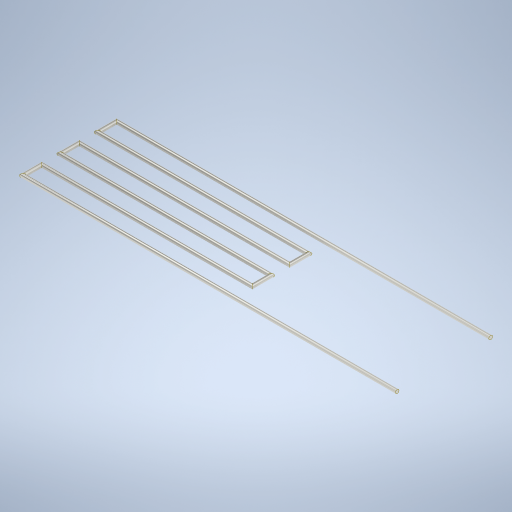
# Autodesk Inventor part: strain guage abs
Saved by Autodesk Inventor 2024.2 (Build 282272000, 272)
## iProperties
Created: 2024-07-17
Part Number: strain guage abs
Material: Silver
Document SubType Name: Modeling
Designer: Makerspace
Density: 10.49 g/cm^3
Appearance: Silver
Author: Makerspace
Autodesk Inventor part; units mm, degrees
ref_plane "XZ Plane" through (0, 0, 0) normal (0, 1, 0) x (-1, 0, 0)
sketch "Sketch1" plane through (0, 0, 0) normal (0, 1, 0) x (-1, 0, 0)
  line L0 (0, 0) -> (38.1, 0)
  line L1 (38.1, 0) -> (38.1, -2.54)
  line L2 (38.1, -2.54) -> (9.525, -2.54)
  line L3 (9.525, -2.54) -> (9.525, -5.08)
  line L4 (9.525, -5.08) -> (38.1, -5.08)
  line L5 (38.1, -5.08) -> (38.1, -7.62)
  line L6 (38.1, -7.62) -> (9.525, -7.62)
  line L7 (9.525, -7.62) -> (9.525, -10.16)
  line L8 (9.525, -10.16) -> (38.1, -10.16)
  line L9 (38.1, -10.16) -> (38.1, -12.7)
  line L10 (38.1, -12.7) -> (9.525, -12.7)
  line L11 (9.525, -12.7) -> (0, -12.7)
  dimension "d0" = 38.1
  dimension "d1" = 2.54
  dimension "d2" = 28.575
  dimension "d3" = 2.54
  constraints: 24 end point, 4 horizontal, 3 perpendicular, 3 point on line, 3 vertical, 2 collinear, 1 parallel
  measures "d0" distance of L0.start L0.end
  measures "d1" distance of L0.end L1.end
  measures "d2" distance of L1.end L2.end
  measures "d3" distance of L2.end L3.end
sketch "Sketch2" plane through (0, 0, 0) normal (1, 0, 0) x (0, 1, 0)
  line L0 (0.635, 0.635) -> (-0.635, -0.635) construction
  line L1 (-0.635, 0.635) -> (0.635, -0.635) construction
  circle A0 centre (0, 0) radius 0.254
  dimension "d4" = 1.27
  dimension "d5" = 1.27
  dimension "d8" = 0.508
  constraints: 4 end point, 2 midpoint, 1 centre point, 1 coincident
  measures "d4" distance of L1.end L0.start
  measures "d5" distance of L0.start L1.start
  measures "d8" diameter of A0
sweep "Sweep1" add profiles "Sketch2" path "Sketch1"
ref_plane "Work Plane1" through (6.35, 0, 0) normal (1, 0, 0) x (0, 1, 0)
ref_plane "Work Plane2" through (0, 0, -6.35) normal (0, 0, 1) x (1, 0, 0)
sketch "Sketch5" plane through (0, 0, 0) normal (1, 0, 0) x (0, 0, -1)
  circle A0 centre (12.7, 0) radius 0.254 projected
  circle A1 centre (12.7, 0) radius 0.254
  circle A2 centre (0, 0) radius 0.254
  constraints: 2 centre point, 2 coincident
extrude "Extrusion3" add sketch "Sketch5" along normal blind 12.7
body "Solid1"
